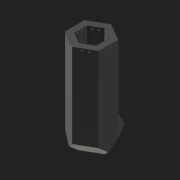
# Autodesk Inventor part: A01
Saved by Autodesk Inventor 2017 (Build 210142000, 142)
## iProperties
Created: 2019-09-19
Part Number: A01
Material: ABS Plastic
Document SubType Name: Modeling
Designer: Dell
Density: 1.06 g/cm^3
Appearance: Smooth - Black
Mass: 2688.13 g
Surface Area: 1514.93 cm^2
Volume: 2535.97 cm^3
Author: Dell
Autodesk Inventor part; units mm, degrees
ref_plane "YZ Plane" through (0, 0, 0) normal (1, 0, 0) x (0, 1, 0)
ref_plane "XZ Plane" through (0, 0, 0) normal (0, 1, 0) x (-1, 0, 0)
ref_plane "XY Plane" through (0, 0, 0) normal (0, 0, 1) x (1, 0, 0)
sketch "Sketch1" plane through (0, 0, 0) normal (0, 0, 1) x (1, 0, 0)
  line L0 (0, 57.735) -> (50, 28.8675)
  line L1 (50, 28.8675) -> (50, -28.8675)
  line L2 (50, -28.8675) -> (0, -57.735)
  line L3 (0, -57.735) -> (-50, -28.8675)
  line L4 (-50, -28.8675) -> (-50, 28.8675)
  line L5 (-50, 28.8675) -> (0, 57.735)
  line L6 (0, 38.1051) -> (33, 19.0526)
  line L7 (33, 19.0526) -> (33, -19.0526)
  line L8 (33, -19.0526) -> (0, -38.1051)
  line L9 (0, -38.1051) -> (-33, -19.0526)
  line L10 (-33, -19.0526) -> (-33, 19.0526)
  line L11 (-33, 19.0526) -> (0, 38.1051)
  point P0 (0, 0)
  point P1 (0, 0)
  dimension "d0" = 100
  dimension "d1" = 66
  constraints: 24 end point, 1 coincident, 1 vertical alignment, 18 other
  measures "d0" distance between parallel lines of L1 L4
  measures "d1" distance between parallel lines of L7 L10
extrude "Extrusion1" add sketch "Sketch1" along normal blind 250
sketch "Sketch2" plane through (50, -28.8675, 0) normal (1, 0, 0) x (0, 0, -1)
  line L0 (-243.5, 21.3675) -> (-243.5, 36.3675) construction
  line L1 (-250, 0) -> (-250, 57.735) projected
  circle A0 centre (-243.5, 36.3675) radius 2.5
  circle A1 centre (-243.5, 21.3675) radius 2.5
  point P0 (0, 28.8675)
  point P1 (-243.5, 28.8675)
  point P2 (-250, 28.8675)
  dimension "d4" = 15
  dimension "d5" = 6.5
  dimension "d6" = 5
  dimension "d7" = 5
  constraints: 2 centre point, 2 coincident, 2 end point, 2 midpoint, 1 horizontal alignment, 1 vertical
  measures "d4" distance of L0.start L0.end
  measures "d5" distance between parallel lines of L0 L1
  measures "d6" diameter of A0
  measures "d7" diameter of A1
extrude "Extrusion2" cut sketch "Sketch2" against normal blind 30
pattern_circular "Circular Pattern1" count 6 over 360 about axis through (0, 0, -10) along (0, 0, 1) of "Extrusion2"
sketch "Sketch8" plane through (-50, 28.8675, 250) normal (-0.5, 0.8660254, 0) x (0.8660254, 0.5, 0)
  line L0 (47.9201, 250) -> (9.815, 250) projected
  line L1 (-28.8675, 250) -> (0, 250) projected
  line L2 (-28.8675, 250) -> (0, 300)
  line L3 (0, 300) -> (57.735, 300)
  line L4 (57.735, 300) -> (86.6025, 250)
  line L5 (86.6025, 250) -> (57.735, 200)
  line L6 (57.735, 200) -> (0, 200)
  line L7 (0, 200) -> (-28.8675, 250)
  point P0 (28.8675, 250)
  constraints: 12 end point, 1 midpoint, 13 other
extrude "Extrusion6" add sketch "Sketch8" against normal up to surface (100 mm away) from surface at 0
sketch "Sketch9" plane through (0, 0, 250) normal (0, 0, 1) x (1, 0, 0)
  line L0 (-50, -28.8675) -> (0, -57.735) projected
  line L1 (-25, -72.1688) -> (-50, -28.8675) projected
  line L2 (-25, -72.1688) -> (0, -57.735) projected
  line L3 (50, -28.8675) -> (50, 28.8675) projected
  line L4 (50, -28.8675) -> (75, -14.4338) projected
  line L5 (50, 28.8675) -> (75, -14.4338) projected
  point P0 (0, 0)
extrude "Extrusion7" cut sketch "Sketch9" against normal through all
sketch "Sketch10" plane through (-50, 28.8675, 250) normal (-0.5, 0.8660254, 0) x (0.8660254, 0.5, 0)
  line L0 (-8.0829, 250) -> (10.3923, 282)
  line L1 (10.3923, 282) -> (47.3427, 282)
  line L2 (47.3427, 282) -> (65.8179, 250)
  line L3 (65.8179, 250) -> (47.3427, 218)
  line L4 (47.3427, 218) -> (10.3923, 218)
  line L5 (10.3923, 218) -> (-8.0829, 250)
  line L6 (0, 300) -> (57.735, 300) projected
  point P0 (28.8675, 250)
  point P1 (28.8675, 250)
  point P2 (28.8675, 282)
  point P3 (28.8675, 300)
  dimension "d32" = 64
  constraints: 12 end point, 2 midpoint, 1 coincident, 1 vertical alignment, 13 other
  measures "d32" distance between parallel lines of L1 L4
extrude "Extrusion8" add sketch "Sketch10" along normal blind 13
sketch "Sketch11" plane through (-56.5, 40.1258, 250) normal (-0.5, 0.8660254, 0) x (0.8660254, 0.5, 0)
  circle A0 centre (28.8675, 250) radius 12.5
  dimension "d35" = 25
  constraints: 1 centre point, 1 coincident
  measures "d35" diameter of A0
extrude "Extrusion9" cut sketch "Sketch11" against normal blind 69.5
sketch "Sketch13" plane through (-33, -0.5774, 50) normal (0, 0, 1) x (1, 0, 0)
  line L0 (0, 0) -> (0, 19.6299) projected
  line L1 (0, 0) -> (16, -27.7128) projected
  line L2 (33, -37.5278) -> (16, -27.7128) projected
  line L3 (66, -18.4752) -> (33, -37.5278) projected
  line L4 (66, 1.1547) -> (66, -18.4752) projected
  line L5 (50, 28.8675) -> (66, 1.1547) projected
  line L6 (33, 38.6825) -> (50, 28.8675) projected
  line L7 (0, 19.6299) -> (33, 38.6825) projected
  line L8 (50, 28.8675) -> (66, 19.6299) projected
  line L9 (50, 28.8675) -> (66, 1.1547) projected
  line L10 (66, 19.6299) -> (66, 1.1547) projected
  line L11 (0, -18.4752) -> (0, 0) projected
  line L12 (16, -27.7128) -> (0, -18.4752) projected
  line L13 (0, 0) -> (16, -27.7128) projected
  point P0 (33, 0.5774)
extrude "Extrusion11" cut sketch "Sketch13" against normal blind 56.5
chamfer "Chamfer1" distance 50 angle 45 1 edges at (25, -43.3013, -50)
body "Solid1"
